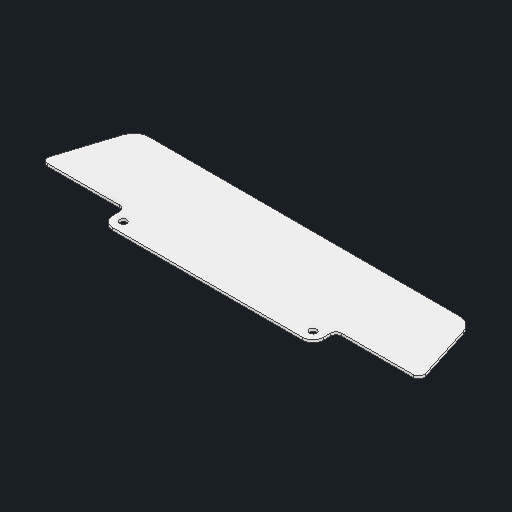
# Autodesk Inventor part: intake_wedge
Saved by Autodesk Inventor 2025 (Build 290162000, 162)
## iProperties
Created: 2024-07-02
Part Number: intake_wedge
Material: Acetal Resin, White
Document SubType Name: Sheet Metal
Designer: Averey Ku
Density: 1.425 g/cm^3
Appearance: Smooth - White
Flat Pattern Width: 5.83184 cm
Flat Pattern Length: 22.6675 cm
Flat Pattern Area: 132.193 cm^2
Sheet Metal Rule: Default_mm
Sheet Metal Width: 2.296 in
Sheet Metal Length: 8.924 in
Sheet Metal Area: 20.490 in^2
Author: Averey Ku
Autodesk Inventor part; units mm, degrees
ref_plane "YZ Plane" through (0, 0, 0) normal (1, 0, 0) x (0, 1, 0)
ref_plane "XZ Plane" through (0, 0, 0) normal (0, 1, 0) x (-1, 0, 0)
ref_plane "XY Plane" through (0, 0, 0) normal (0, 0, 1) x (1, 0, 0)
sketch "main" plane through (0, 0, 0) normal (0, 0, 1) x (1, 0, 0)
  line L0 (-49.2738, 43.4655) -> (65.0262, 43.4655)
  circle A0 centre (65.0262, 37.1155) radius 2.1844
  line L1 (71.3762, 37.1155) -> (71.3762, 32.7721)
  arc A1 (71.3762, 37.1155) -> (65.0262, 43.4655) centre (65.0262, 37.1155) ccw
  line L2 (-71.4988, 29.5971) -> (-102.2861, 29.5971)
  line L3 (-105.3112, 25.4581) -> (-94.5785, -8.22)
  line L4 (-58.7988, 29.5971) -> (118.0384, 29.5971)
  line L5 (121.0635, 25.4581) -> (110.3309, -8.22)
  line L6 (101.2556, -14.8529) -> (-85.5032, -14.8529)
  arc A2 (-94.5785, -8.22) -> (-85.5032, -14.8529) centre (-85.5032, -5.3279) ccw
  arc A3 (101.2556, -14.8529) -> (110.3309, -8.22) centre (101.2556, -5.3279) ccw
  arc A4 (-102.2861, 29.5971) -> (-105.3112, 25.4581) centre (-102.2861, 26.4221) ccw
  arc A5 (121.0635, 25.4581) -> (118.0384, 29.5971) centre (118.0384, 26.4221) ccw
  arc A6 (71.3762, 32.7721) -> (74.5512, 29.5971) centre (74.5512, 32.7721) ccw
  line L7 (-58.7988, 29.5971) -> (-71.4988, 29.5971)
  circle A7 centre (-49.2738, 37.1155) radius 2.1844
  arc A8 (-49.2738, 43.4655) -> (-55.6238, 37.1155) centre (-49.2738, 37.1155) ccw
  line L8 (-55.6238, 37.1155) -> (-55.6238, 32.7721)
  arc A9 (-58.7988, 29.5971) -> (-55.6238, 32.7721) centre (-58.7988, 32.7721) ccw
  point P0 (1.5262, 9.2461)
  point P1 (-55.8302, 29.5971)
  point P2 (-106.6302, 29.5971)
  point P3 (-92.4647, -14.8529)
  point P4 (122.3826, 29.5971)
  point P5 (108.2171, -14.8529)
  dimension "d0" = 12.7
  dimension "d11" = 50.8
  dimension "d17" = 9.525
  dimension "d18" = 9.525
  dimension "d19" = 3.175
  dimension "d20" = 3.175
  dimension "d23" = 44.45
  dimension "d24" = 4.3688
  dimension "d25" = 186.7588
  dimension "d26" = 3.175
  measures "d0" diameter of A1
  measures "d11" distance of point (-55.83, 29.597) point (-106.63, 29.597)
  measures "d17" radius of A2
  measures "d18" radius of A3
  measures "d19" radius of A4
  measures "d20" radius of A6
  measures "d23" distance between parallel lines of L6 L7
  measures "d24" diameter of A7
  measures "d25" distance of L6.start L6.end
  measures "d26" radius of A9
sketch "Sketch1" plane through (0, 0, 0) normal (0, 1, 0) x (-1, 0, 0)
  line L0 (-114.3, 6.35) -> (0, 6.35)
  circle A0 centre (0, 0) radius 2.1844
  line L1 (6.35, 0) -> (6.35, -4.3434)
  arc A1 (6.35, 0) -> (0, 6.35) centre (0, 0) ccw
  line L2 (-136.525, -7.5184) -> (-167.3123, -7.5184)
  line L3 (-170.3374, -11.6575) -> (-159.6047, -45.3356)
  line L4 (-123.825, -7.5184) -> (53.0123, -7.5184)
  line L5 (56.0374, -11.6575) -> (45.3047, -45.3356)
  line L6 (36.2294, -51.9684) -> (-150.5294, -51.9684)
  arc A2 (-159.6047, -45.3356) -> (-150.5294, -51.9684) centre (-150.5294, -42.4434) ccw
  arc A3 (36.2294, -51.9684) -> (45.3047, -45.3356) centre (36.2294, -42.4434) ccw
  arc A4 (-167.3123, -7.5184) -> (-170.3374, -11.6575) centre (-167.3123, -10.6934) ccw
  arc A5 (56.0374, -11.6575) -> (53.0123, -7.5184) centre (53.0123, -10.6934) ccw
  arc A6 (6.35, -4.3434) -> (9.525, -7.5184) centre (9.525, -4.3434) ccw
  line L7 (-123.825, -7.5184) -> (-136.525, -7.5184)
  circle A7 centre (-114.3, 0) radius 2.1844
  arc A8 (-114.3, 6.35) -> (-120.65, 0) centre (-114.3, 0) ccw
  line L8 (-120.65, 0) -> (-120.65, -4.3434)
  arc A9 (-123.825, -7.5184) -> (-120.65, -4.3434) centre (-123.825, -4.3434) ccw
  constraints: 1 other
extrude "Extrusion1" add sketch "Sketch1" along normal blind 1.5875
feature "Bend Part2" [suppressed]
equation "\"BendRadius\" = Thickness"
equation "\"BendReliefWidth\" = Thickness"
equation "\"BendReliefDepth\" = 0.5 * Thickness"
equation "\"CornerReliefSize\" = 4 * Thickness"
equation "\"MinimumRemnant\" = 2 * Thickness"
equation "\"TransitionRadius\" = BendRadius"
equation "\"JacobiRadiusSize\" = BendRadius"
equation "\"GapSize\" = Thickness"
equation "\"Thickness\" = 1.5875"
body "Solid1"
